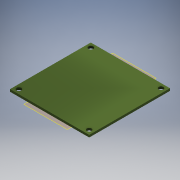
# Autodesk Inventor part: Crusher_Board
Saved by Autodesk Inventor 2016 (Build 200138000, 138)
## iProperties
Created: 2016-04-23
Part Number: Crusher_Board
Material: Generic
Document SubType Name: Modeling
Designer: 3DPrinterUser
Density: 1 g/cm^3
Appearance: Olive Green
Author: 3DPrinterUser
Autodesk Inventor part; units mm, degrees
ref_plane "YZ Plane" through (0, 0, 0) normal (1, 0, 0) x (0, 1, 0)
ref_plane "XZ Plane" through (0, 0, 0) normal (0, 1, 0) x (-1, 0, 0)
ref_plane "XY Plane" through (0, 0, 0) normal (0, 0, 1) x (1, 0, 0)
ref_plane "Work Plane1" through (0, 0, 0) normal (0, 0, 1) x (1, 0, 0)
sketch "Sketch1" plane through (0, 0, 0) normal (0, 0, 1) x (1, 0, 0)
  circle A0 centre (-3, -23) radius 1.55 projected
  circle A1 centre (-49.9646, -23) radius 1.55 projected
  circle A2 centre (-49.9646, -71) radius 1.55 projected
  circle A3 centre (-3, -71) radius 1.55 projected
  line L0 (0, -74) -> (-52.9646, -74) projected
  line L1 (0, -20) -> (0, -74) projected
  line L2 (0, -20) -> (-52.9646, -20) projected
  line L3 (-52.9646, -20) -> (-52.9646, -74) projected
  point P0 (0, 0)
extrude "Extrusion1" add sketch "Sketch1" along normal blind 1.5
body "Solid1"
